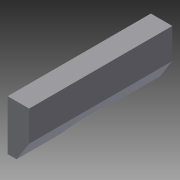
# Autodesk Inventor part: ShooterFrontMount
Saved by Autodesk Inventor 2014 (Build 180170000, 170)
## iProperties
Created: 2016-02-03
Part Number: ShooterFrontMount
Material: Generic
Document SubType Name: Modeling
Designer: zoldberg
Density: 1 g/cm^3
Appearance: Default
Author: zoldberg
Autodesk Inventor part; units mm, degrees
ref_plane "YZ Plane" through (0, 0, 0) normal (1, 0, 0) x (0, 1, 0)
ref_plane "XZ Plane" through (0, 0, 0) normal (0, 1, 0) x (-1, 0, 0)
ref_plane "XY Plane" through (0, 0, 0) normal (0, 0, 1) x (1, 0, 0)
sketch "Sketch1" plane through (0, 0, 0) normal (0, 0, 1) x (1, 0, 0)
  line L0 (19.05, -44.45) -> (-19.05, -44.45)
  line L1 (-19.05, -44.45) -> (-19.05, 44.45)
  line L2 (-19.05, 44.45) -> (19.05, 44.45)
  line L3 (19.05, 44.45) -> (19.05, -44.45)
  line L4 (19.05, -44.45) -> (-19.05, 44.45) construction
  line L5 (-19.05, -44.45) -> (19.05, 44.45) construction
  point P0 (0, 0)
  dimension "d0" = 38.1
  dimension "d1" = 88.9
  constraints: 12 end point, 2 midpoint, 2 parallel, 1 horizontal, 1 perpendicular
  measures "d0" distance of L1.end L2.end
  measures "d1" distance of L2.end L0.start
extrude "Extrusion1" add sketch "Sketch1" along normal blind 254
sketch "Sketch2" plane through (0, 0, 254) normal (0, 0, 1) x (1, 0, 0)
  line L0 (-19.05, -44.45) -> (19.05, -44.45) projected
  line L1 (19.05, -44.45) -> (19.05, 44.45) projected
  line L2 (-3.175, -44.45) -> (19.05, -9.525)
  point P0 (0, 0)
  dimension "d7" = 22.225
  dimension "d8" = 34.925
  constraints: 2 end point, 2 point on line
  measures "d7" distance of L2.start L0.end
  measures "d8" distance of L2.end L0.end
extrude "Extrusion2" cut sketch "Sketch2" against normal blind 254
sketch "Sketch3" plane through (-19.05, -44.45, 0) normal (-1, 0, 0) x (0, 0, 1)
  line L0 (0, 0) -> (254, 0) projected
  arc A0 (177.8, 0) -> (76.2, 0) centre (127, -116.3974) ccw
  point P0 (0, 44.45)
  dimension "d11" = 76.2
  dimension "d12" = 76.2
  dimension "d13" = 127
  constraints: 2 point on circle, 2 point on line, 1 centre point
  measures "d11" distance of L0.start A0.end
  measures "d12" distance of L0.end A0.start
  measures "d13" radius of A0
extrude "Extrusion3" cut sketch "Sketch3" against normal blind 254
equation "\"d12\" = d11"
body "Solid1"
